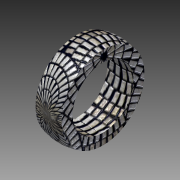
# Autodesk Inventor part: bigWheelMosaic
Saved by Autodesk Inventor 2013 (Build 170138000, 138)
## iProperties
Created: 2013-01-08
Part Number: bigWheelMosaic
Material: Generic
Document SubType Name: Modeling
Designer: Nano
Density: 1 g/cm^3
Author: Nano
Autodesk Inventor part; units mm, degrees
ref_plane "YZ Plane" through (0, 0, 0) normal (1, 0, 0) x (0, 1, 0)
ref_plane "XZ Plane" through (0, 0, 0) normal (0, 1, 0) x (-1, 0, 0)
ref_plane "XY Plane" through (0, 0, 0) normal (0, 0, 1) x (1, 0, 0)
sketch "Sketch1" plane through (0, 0, 0) normal (0, 0, 1) x (1, 0, 0)
  line L0 (-38.1, 0) -> (38.1, 0)
  line L1 (38.1, 0) -> (38.1, 38.1)
  line L2 (38.1, 38.1) -> (-38.1, 38.1)
  line L3 (-38.1, 38.1) -> (-38.1, 0)
  circle A0 centre (0, -88.9) radius 127
  line L4 (0, -88.9) -> (-189.5771, -88.9) construction
  point P0 (0, 0)
  point P1 (-38.1, 32.2503)
  point P2 (38.1, 32.2503)
  dimension "d0" = 76.2
  dimension "d1" = 38.1
  dimension "d2" = 38.1
  dimension "d3" = 127
  constraints: 10 end point, 2 parallel, 2 perpendicular, 2 point on circle, 2 point on line, 1 centre point, 1 coincident, 1 horizontal, 1 tangent
  measures "d0" distance of L2.end L1.end
  measures "d1" distance of L1.end L0.end
  measures "d2" distance of L0.start point (0, 0)
  measures "d3" distance from line of L2 point (0, -88.9)
revolve "Revolution1" add sketch "Sketch1" angle 360 about axis through (0, -88.9, 0) along (-1, 0, 0) picked at (0, 12.7) contours L3 A0 L1 L0
equation "\"d2\" = 0.5 * d0"
body "Solid1"
